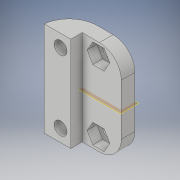
# Autodesk Inventor part: x_carriage_aio_ir_probe
Saved by Autodesk Inventor 2019 (Build 230136000, 136)
## iProperties
Created: 2019-11-10
Part Number: x_carriage_aio_ir_probe
Material: Generisch
Document SubType Name: Modeling
Designer: marc
Density: 1 g/cm^3
Appearance: Vorgabe
Author: marc
## iProperties of the stored document x_carriage_aio_ir_probe_3D-Druck.ipt
Created: 2019-11-10
Part Number: x_carriage_aio_ir_probe_3D-Druck
Material: Generisch
Document SubType Name: Modeling
Designer: marc
Density: 1 g/cm^3
Appearance: Vorgabe
Author: marc
Autodesk Inventor part; units mm, degrees
ref_plane "YZ Plane" through (0, 0, 0) normal (1, 0, 0) x (0, 1, 0)
ref_plane "XZ Plane" through (0, 0, 0) normal (0, 1, 0) x (-1, 0, 0)
ref_plane "XY Plane" through (0, 0, 0) normal (0, 0, 1) x (1, 0, 0)
derived "x_carriage_aio_base.ipt"
sketch "Skizze37" plane through (-7.3074, 55, 2.4) normal (0, 0, 1) x (1, 0, 0)
  circle A0 centre (4.3074, -36.7) radius 1.7
  circle A1 centre (4.3074, -18.3) radius 1.7
  circle A2 centre (11.3074, -18.3) radius 1.55
  circle A3 centre (11.3074, -36.7) radius 1.55
  arc A4 (17.3074, -20.75) -> (11.5574, -15) centre (11.5574, -20.75) ccw
  line L0 (7.3074, -15) -> (11.5574, -15)
  line L1 (0, -15) -> (7.3074, -15)
  line L2 (0, -40) -> (0, -15)
  line L3 (7.3074, -40) -> (0, -40)
  line L4 (7.3074, -40) -> (11.5574, -40)
  arc A5 (11.5574, -40) -> (17.3074, -34.25) centre (11.5574, -34.25) ccw
  line L5 (17.3074, -20.75) -> (17.3074, -34.25)
  line L6 (7.3074, -15) -> (2.3074, -15)
  line L7 (0, -15) -> (2.3074, -15)
  point P0 (7.3074, -55)
extrude "Extrusion1" add sketch "Skizze37" along normal blind 3.6
sketch "Skizze2" plane through (-7.3074, 40, 6) normal (0, 0, 1) x (1, 0, 0)
  circle A0 centre (11.3074, -21.7) radius 1.55 projected
  line L0 (9.8074, -24.2981) -> (8.3074, -21.7)
  line L1 (8.3074, -21.7) -> (9.8074, -19.1019)
  line L2 (9.8074, -19.1019) -> (12.8074, -19.1019)
  line L3 (12.8074, -19.1019) -> (14.3074, -21.7)
  line L4 (14.3074, -21.7) -> (12.8074, -24.2981)
  line L5 (12.8074, -24.2981) -> (9.8074, -24.2981)
  line L6 (0, -25) -> (11.5574, -25) projected
  point P0 (7.3074, -40)
  point P1 (11.3074, -21.7)
  dimension "d3" = 3
  constraints: 12 end point, 1 coincident, 1 parallel, 13 other
  measures "d3" distance of L4.end L0.start
extrude "Extrusion2" cut sketch "Skizze2" against normal blind 2.6
ref_plane "Arbeitsebene2" through (-7.3074, 27.5, 2.4) normal (0, 1, 0) x (1, 0, 0)
mirror "Spiegeln1" about plane through (-7.3074, 27.5, 2.4) normal (0, 1, 0) of "Extrusion2"
sketch "Skizze3" plane through (-7.3074, 40, 6) normal (0, 0, 1) x (1, 0, 0)
  circle A0 centre (4.3074, -21.7) radius 1.7 projected
  line L0 (1.4574, -23.3454) -> (1.4574, -20.0546)
  line L1 (1.4574, -20.0546) -> (4.3074, -18.4091)
  line L2 (4.3074, -18.4091) -> (7.1574, -20.0546)
  line L3 (7.1574, -20.0546) -> (7.1574, -23.3454)
  line L4 (7.1574, -23.3454) -> (4.3074, -24.9909)
  line L5 (4.3074, -24.9909) -> (1.4574, -23.3454)
  line L6 (0, 0) -> (0, -25) projected
  point P0 (7.3074, -40)
  dimension "d7" = 5.7
  constraints: 12 end point, 1 coincident, 1 parallel, 13 other
  measures "d7" distance between parallel lines of L0 L3
extrude "Extrusion3" [suppressed]
sketch "Skizze5" plane through (-7.3074, 40, 6) normal (0, 0, 1) x (1, 0, 0)
  line L0 (7, 0) -> (7, -25)
  line L1 (0, 0) -> (0, -25) projected
  circle A0 centre (4.3074, -21.7) radius 1.7 projected
  circle A1 centre (4.3074, -3.3) radius 1.7 projected
  line L2 (11.5574, 0) -> (0, 0) projected
  line L3 (0, -25) -> (11.5574, -25) projected
  point P0 (7.3074, -40)
  dimension "d16" = 7
  constraints: 2 end point, 2 point on line, 1 vertical
  measures "d16" distance between parallel lines of L1 L0
extrude "Extrusion5" add sketch "Skizze5" along normal blind 3
fillet "Rundung1" radius 7.5 1 edges at (-7.3074, 27.5, 2.4)
